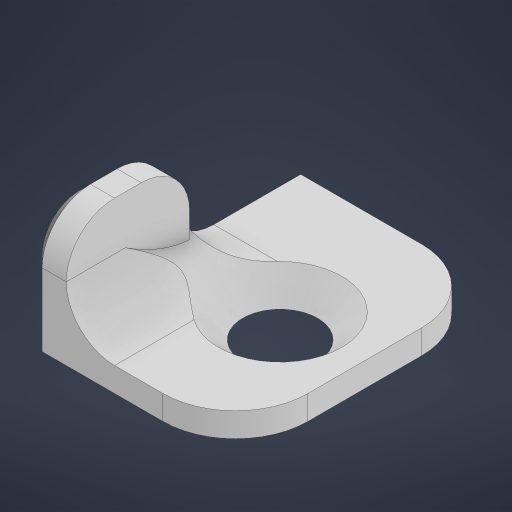
# Autodesk Inventor part: mocowanie_tofa
Saved by Autodesk Inventor 2024 (Build 280153000, 153)
## iProperties
Created: 2024-05-24
Part Number: mocowanie_tofa
Material: Generic
Document SubType Name: Modeling
Designer: Adam
Density: 1 g/cm^3
Appearance: Default
Mass: 0.10087 g
Surface Area: 2.61074 cm^2
Volume: 0.10087 cm^3
Author: Adam
Autodesk Inventor part; units mm, degrees
ref_plane "YZ Plane" through (0, 0, 0) normal (1, 0, 0) x (0, 1, 0)
ref_plane "XZ Plane" through (0, 0, 0) normal (0, 1, 0) x (-1, 0, 0)
ref_plane "XY Plane" through (0, 0, 0) normal (0, 0, 1) x (1, 0, 0)
sketch "Sketch1" plane through (0, 0, 0) normal (0, 0, 1) x (1, 0, 0)
  line L0 (0, 0) -> (8, 0)
  line L1 (8, 0) -> (8, 1)
  line L2 (8, 1) -> (1, 1)
  line L3 (1, 1) -> (1, 5)
  line L4 (1, 5) -> (0, 5)
  line L5 (0, 5) -> (0, 0)
  dimension "d0" = 8
  dimension "d1" = 5
  dimension "d2" = 1
  dimension "d8" = 1
  constraints: 12 end point, 5 perpendicular, 1 horizontal
  measures "d0" distance between parallel lines of L1 L5
  measures "d1" distance of L4.end L0.start
  measures "d2" distance between parallel lines of L2 L0
  measures "d8" distance between parallel lines of L3 L5
extrude "Extrusion1" add sketch "Sketch1" along normal blind 10.7
sketch "Sketch3" plane through (1, 1, 0) normal (0, 1, 0) x (1, 0, 0)
  line L0 (7, 0) -> (7, -10.7) projected
  line L1 (7, -10.7) -> (0, -10.7) projected
  point P0 (-1, 0)
  point P1 (3.5, -5.35)
  point P2 (3.5, -10.7)
  dimension "d11" = 3.5
  dimension "d12" = 5.35
  constraints: 1 midpoint
  measures "d11" distance from line of point (3.5, -5.35) L0
  measures "d12" distance of point (3.5, -10.7) point (3.5, -5.35)
hole "Hole1" at (4.5, 1, 5.35) direction (0, -1, 0) diameter 3.1 end through all
fillet "Fillet1" radius 3 2 edges at (8, 0.5, 0) (8, 0.5, 10.7)
chamfer "Chamfer2" distance 1 angle 45 1 edges at (4.5, 1, 3.8) measured on face at (4.5, 1, 3.3)
sketch "Sketch6" plane through (0, 0, 0) normal (-1, 0, 0) x (0, 0, 1)
  line L0 (0, 5) -> (10.7, 5) projected
  line L1 (10.7, 5) -> (10.7, 0) projected
  circle A0 centre (8.15, 2.45) radius 1.55
  point P0 (0, 0)
  point P1 (10.7, 2.5)
  dimension "d39" = 2.55
  dimension "d40" = 2.55
  dimension "d41" = 3.1
  constraints: 1 centre point, 1 coincident, 1 midpoint
  measures "d39" distance from line of L0 point (8.15, 2.45)
  measures "d40" horizontal distance of point (10.7, 2.5) point (8.15, 2.45)
  measures "d41" diameter of A0
extrude "Extrusion5" add sketch "Sketch6" along normal blind 1
sketch "Sketch7" plane through (0, 0, 0) normal (-1, 0, 0) x (0, 0, 1)
  line L0 (0, 5) -> (10.7, 5) projected
  line L1 (3, 1) -> (7.7, 1) projected
  line L2 (0, 5) -> (5.6, 5)
  line L3 (5.6, 5) -> (5.6, 1)
  line L4 (5.6, 1) -> (0, 1)
  line L5 (0, 1) -> (0, 5)
  point P0 (0, 0)
  dimension "d44" = 5.6
  constraints: 8 end point, 2 parallel, 1 horizontal, 1 perpendicular, 1 point on line
  measures "d44" distance of L3.end L4.end
extrude "Extrusion6" cut sketch "Sketch7" against normal blind 1
fillet "Fillet5" radius 2 4 edges at (0.5, 5, 5.6) (0.5, 5, 10.7) (0.5, 1, 5.6) (1, 1, 8.15)
body "Solid1"
